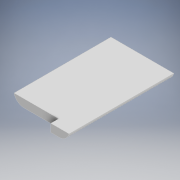
# Autodesk Inventor part: Case_Cover
Saved by Autodesk Inventor 2020 (Build 240168000, 168)
## iProperties
Created: 2019-11-07
Part Number: Case_Cover
Material: 일반
Document SubType Name: Modeling
Designer: Knowblesse
Density: 1 g/cm^3
Appearance: 기본값
Author: Knowblesse
## iProperties of the stored document _3D 인쇄.ipt
Created: 2019-11-07
Part Number: _3D 인쇄
Material: 일반
Document SubType Name: Modeling
Designer: Knowblesse
Density: 1 g/cm^3
Appearance: 기본값
Author: Knowblesse
Autodesk Inventor part; units mm, degrees
ref_plane "YZ Plane" through (0, 0, 0) normal (1, 0, 0) x (0, 1, 0)
ref_plane "XZ Plane" through (0, 0, 0) normal (0, 1, 0) x (-1, 0, 0)
ref_plane "XY Plane" through (0, 0, 0) normal (0, 0, 1) x (1, 0, 0)
sketch "스케치1" plane through (0, 0, 0) normal (0, 1, 0) x (-1, 0, 0)
  line L0 (0, 0) -> (12, 0)
  line L1 (12, 0) -> (12, -20)
  line L2 (12, -20) -> (0, -20)
  line L3 (0, -20) -> (0, 0)
  dimension "d0" = 12
  dimension "d1" = 20
  constraints: 8 end point, 2 parallel, 1 horizontal, 1 perpendicular
  measures "d0" distance of L1.end L2.end
  measures "d1" distance of L0.end L1.end
extrude "돌출1" add sketch "스케치1" along normal blind 1.5
fillet "모깎기1" radius 2 2 edges at (-12, 0, -10) (0, 0, -10)
sketch "스케치3" plane through (-10.0635, 0, 0) normal (0, 0, 1) x (1, 0, 0)
  arc A0 (8.127, 0) -> (10.0635, 1.5) centre (8.127, 2) ccw projected
  line L0 (-1.9365, 1.5) -> (10.0635, 1.5) projected
  arc A1 (-1.9365, 1.5) -> (0, 0) centre (0, 2) ccw projected
  line L1 (0, 0) -> (8.127, 0) projected
  line L2 (6.5635, 0) -> (6.5635, 1.5)
  line L3 (-1.9365, 1.5) -> (10.0635, 1.5) projected
  point P0 (10.0635, 0)
  dimension "d15" = 3.5
  constraints: 2 end point, 2 point on line, 1 perpendicular
  measures "d15" distance from line of L2 L0.end
extrude "돌출3" cut sketch "스케치3" against normal blind 1.5 contours L1 A1 L0 L2
